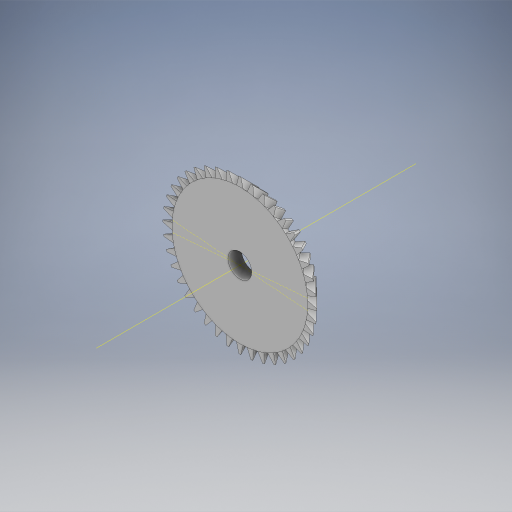
# Autodesk Inventor part: big gear
Saved by Autodesk Inventor 2024 (Build 280153000, 153)
## iProperties
Created: 2024-04-10
Part Number: big gear
Material: Generic
Document SubType Name: Modeling
Designer: Alex
Density: 1 g/cm^3
Appearance: Default
Author: Alex
Autodesk Inventor part; units mm, degrees
sketch "Sketch1" plane through (0, 0, 0) normal (0, 1, 0) x (-1, 0, 0)
  line L0 (0, 0) -> (-40, 0) construction
  line L1 (-40, 0) -> (-32, -8)
  line L2 (-32, -8) -> (-7, -8)
  line L3 (0, 0) -> (0, -8) construction
  line L4 (-7, 0) -> (-7, -8)
  line L5 (-7, -8) -> (0, -8) construction
  line L6 (-40, 0) -> (-7, 0)
  dimension "d0" = 40
  dimension "d1" = 45
  dimension "d2" = 8
  dimension "d3" = 7
  constraints: 14 end point, 3 horizontal, 2 perpendicular, 1 coincident, 1 collinear, 1 point on line, 1 vertical
  measures "d0" distance of L0.start L0.end
  measures "d1" angle of L0 L1
  measures "d2" distance between parallel lines of L0 L2
  measures "d3" distance between parallel lines of L3 L4
revolve "Revolution1" add sketch "Sketch1" angle 360 about axis through (0, 0, 0) along (0, 0, -1)
ref_plane "Work Plane1" through (0, 0, 0) normal (0.0795, 0.9968, 0) x (0, 0, 1)
ref_plane "Work Plane2" through (0, 0, 0) normal (-0.0795, 0.9968, 0) x (0, 0, 1)
sketch "Sketch2" plane through (0, 0, 0) normal (-0.0795, 0.9968, 0) x (0, 0, 1)
  line L0 (0, 40) -> (0, -40) construction
  line L1 (-8, 32) -> (-8, -32) construction
  line L2 (-8, -32) -> (0, -40) construction
  point P0 (0, 0)
  constraints: 2 end point
sketch "Sketch3" plane through (0, 0, 0) normal (0.0795, 0.9968, 0) x (0, 0, 1)
  line L0 (0, 40) -> (0, -40) construction
  line L1 (-8, 32) -> (-8, -32) construction
  line L2 (0, -40) -> (-8, -32) construction
  line L3 (0, -40) -> (-8, -32) construction
  point P0 (0, 0)
  constraints: 2 end point, 1 collinear
ref_plane "Work Plane5" through (-31.8986, 2.5455, -8) normal (-0.706, 0, 0.7082) x (0, 1, 0)
ref_plane "Work Plane4" through (0, 0, 0) normal (-0.706, 0, 0.7082) x (0, 1, 0)
sketch "Sketch4" plane through (-31.8986, 2.5455, -8) normal (-0.706, 0, 0.7082) x (0, 1, 0)
  line L0 (0, 0) -> (-5.091, 0) construction
  ellipse E0 centre (-2.5455, -28.2394) end of major axis (-42.5455, -28.2394) minor radius 28.3291 projected
  line L1 (0, 0) -> (-1.0919, 3) construction
  line L2 (-1.0919, 3) -> (-3.9991, 3) construction
  line L3 (-3.9991, 3) -> (-5.091, 0) construction
  line L4 (-2.5455, 3) -> (-2.5455, 0) construction
  line L5 (-0.565, 0) -> (-1.9805, 3.889)
  line L6 (-1.9805, 3.889) -> (-3.1105, 3.889)
  line L7 (-3.1105, 3.889) -> (-4.526, 0)
  line L8 (-0.565, 0) -> (-4.526, 0)
  line L9 (-2.5455, 3.889) -> (-2.5455, 0) construction
  line L10 (-2.5455, 3) -> (-2.5455, 0) construction
  point P0 (-2.5455, -28.2394)
  point P1 (-5.079, 0.0329)
  point P2 (-0.012, 0.0329)
  point P3 (-4.5057, 0.0557)
  point P4 (-0.5853, 0.0557)
  dimension "d8" = 3
  dimension "d9" = 70
  dimension "d15" = 1.13
  dimension "d16" = 0.565
  constraints: 22 end point, 4 midpoint, 3 parallel, 2 horizontal, 2 vertical, 1 perpendicular, 1 other
  measures "d8" distance between parallel lines of L0 L2
  measures "d9" angle of L0 L3
  measures "d15" distance of L5.end L6.end
  measures "d16" distance of L0.end L7.end
extrude "Extrusion2" add sketch "Sketch4" along normal up to surface contours E0 L7 L6 L5 surface through (40, 0, 0) normal (0, 0, 1)
pattern_circular "Circular Pattern2" count 40 over 360 about axis through (0, 0, -10) along (0, 0, 1) of "Extrusion2"
ref_plane "Work Plane3" through (-39.8732, 3.1819, 0) normal (-0.7082, 0, -0.706) x (0.7049, -0.0562, -0.7071)
body "Solid1"
